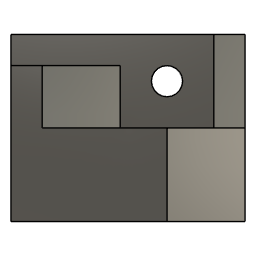
task1 A robocon (Autodesk Fusion 360 design; units mm, degrees)
Autodesk Fusion 360 part; units mm, degrees
sketch "Sketch1" plane through (0, 0, 0) normal (0, 0, 1) x (1, 0, 0)
  line L0 (7.5, 9) -> (-7.5, 9)
  line L1 (-7.5, 9) -> (-7.5, -9)
  line L2 (-7.5, -9) -> (2.5, -9)
  line L3 (7.5, -3) -> (7.5, 7)
  line L4 (2.5, -9) -> (7.5, -3)
  line L5 (5.5, 7) -> (7.5, 9)
  line L6 (7.5, 7) -> (7.5, 9)
  line L7 (5.5, 7) -> (-7.5, 7)
  dimension "d2" = 18
  dimension "d3" = 10
  dimension "d4" = 2
  dimension "d5" = 2
  constraint horizontal L0
  constraint perpendicular L0 L1
  constraint parallel L0 L2
  constraint parallel L1 L3
  constraint perpendicular L0 L6
  constraint coincident L1 L7.end
  constraint perpendicular L1 L7
  measures "d2" distance of L0.end L1.end
  measures "d3" distance of L1.end L2.end
  measures "d4" distance of L0.start L3.end
  measures "d5" distance of L3.end L5.start
extrude "Extrude1" add sketch "Sketch1" along normal blind 6 contours L1 L2 L3 L4 L5 L6 L7
sketch "Sketch2" plane through (0, 0, 6) normal (0, 0, 1) x (-1, 0, 0)
  line L0 (-5.5, -7) -> (7.5, -7)
  line L1 (7.5, -7) -> (7.5, 9)
  line L2 (7.5, 9) -> (-2.5, 9)
  line L3 (-2.5, 9) -> (-7.5, 3)
  line L4 (-7.5, 3) -> (-7.5, -9)
  line L5 (-7.5, -9) -> (-5.5, -7)
  line L6 (-7.5, -9) -> (7.5, -9)
  line L7 (7.5, -9) -> (7.5, -7)
  dimension "d8" = 15
  constraint coincident L4.end L5.start
  constraint perpendicular L4 L6
  constraint coincident L0.end L1.start
  measures "d8" distance of L4.end L6.end
extrude "Extrude2" add sketch "Sketch2" along normal blind 6 and the other way blind 6 contours L0 L5 L6 L7
extrude "Extrude3" add 1 faces at (-2.5, 9, 6) along direction (0, 1, 0) blind 2
sketch "Sketch3" plane through (0, 7, 0) normal (0, -1, 0) x (1, 0, 0)
  line L0 (-7.5, 6) -> (5.5, 6)
  line L1 (5.5, 6) -> (5.5, 12)
  line L2 (5.5, 12) -> (-7.5, 12)
  line L3 (-7.5, 12) -> (-7.5, 6)
  line L4 (5.5, 12) -> (5.5, 10) construction
  line L5 (5.5, 10) -> (-0.5, 10) construction
  line L6 (-0.5, 10) -> (-7.5, 10)
  line L7 (-0.5, 10) -> (-0.5, 6)
  constraint coincident L1.end L2.start
  constraint coincident L1 L4.end
  constraint perpendicular L2 L4
  constraint perpendicular L4 L5
  constraint coincident L3 L6.end
  constraint perpendicular L3 L6
  constraint perpendicular L5 L7
extrude "Extrude4" add sketch "Sketch3" along normal blind 16 contours L0 L3 L6 L7
sketch "Sketch4" plane through (0, 0, 10) normal (0, 0, 1) x (-1, 0, 0)
  line L0 (0.5, -7) -> (7.5, -7)
  line L1 (7.5, -7) -> (7.5, 9)
  line L2 (7.5, 9) -> (0.5, 9)
  line L3 (0.5, 9) -> (0.5, -7)
  line L4 (7.5, 9) -> (5.5, 9)
  line L5 (5.5, 9) -> (5.5, 5)
  line L6 (0.5, -7) -> (0.5, -1)
  line L7 (5.5, 5) -> (0.5, -1)
  dimension "d17" = 2
  dimension "d18" = 6
  constraint coincident L1.end L2.start
  constraint perpendicular L1 L4
  constraint perpendicular L4 L5
  constraint coincident L0.start L3.end
  constraint perpendicular L0 L6
  measures "d17" distance of L1.end L4.end
  measures "d18" distance of L0.start L6.end
extrude "Extrude5" cut sketch "Sketch4" against normal blind 4 contours L2 L3 L5 L7
sketch "Sketch5" plane through (0, 0, 10) normal (0, 0, 1) x (-1, 0, 0)
  line L0 (5.5, 9) -> (5.5, 5)
  line L1 (5.5, 5) -> (0.5, -1)
  line L2 (0.5, -1) -> (0.5, -7)
  line L3 (0.5, -7) -> (7.5, -7)
  line L4 (7.5, -7) -> (7.5, 9)
  line L5 (7.5, 9) -> (5.5, 9)
  line L6 (0.5, -1) -> (7.5, -1) construction
  circle A0 centre (4, -4) radius 1
  dimension "d21" = 2
  constraint coincident L1.end L2.start
  constraint coincident L4 L6.end
  constraint perpendicular L4 L6
  measures "d21" diameter of A0
extrude "Extrude6" cut sketch "Sketch5" against normal blind 6 contours A0
sketch "Sketch6" plane through (0, 7, 0) normal (0, -1, 0) x (1, 0, 0)
  line L0 (-0.5, 10) -> (-0.5, 6)
  line L1 (-0.5, 6) -> (5.5, 6)
  line L2 (5.5, 6) -> (5.5, 12)
  line L3 (5.5, 12) -> (-7.5, 12)
  line L4 (-7.5, 12) -> (-7.5, 10)
  line L5 (-7.5, 10) -> (-0.5, 10)
  line L6 (-0.5, 12) -> (-0.5, 11.8671) construction
  line L7 (-0.5, 11.8671) -> (-0.5, 10) construction
  circle A0 centre (2.5, 9) radius 1
  dimension "d24" = 2
  constraint coincident L3 L6.start
  constraint perpendicular L3 L6
  constraint coincident L0.start L5.end
  constraint perpendicular L5 L7
  measures "d24" diameter of A0
extrude "Extrude7" cut sketch "Sketch6" against normal blind 3.5 contours A0
extrude "Extrude8" cut 1 faces at (2.6218, 10.5, 8.6897) along direction (0, 1, 0) blind 6
extrude "Extrude9" cut 1 faces at (-4.4091, 4.2521, 4) along direction (0, 0, -1) blind 58
